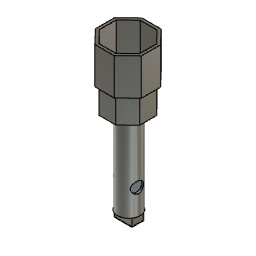
idea2 v1 (Autodesk Fusion 360 design; units mm, degrees)
Autodesk Fusion 360 part; units mm, degrees
sketch "Schizzo1" plane through (0, 0, 0) normal (0, 1, 0) x (1, 0, 0)
  line L0 (-15, -25) -> (15, -25)
  line L1 (15, -25) -> (37.4782, -5.1322)
  line L2 (37.4782, -5.1322) -> (37.4782, 24.8678)
  line L3 (37.4782, 24.8678) -> (15.4232, 45.2044)
  line L4 (15.4232, 45.2044) -> (-14.5768, 45.2044)
  line L5 (-14.5768, 45.2044) -> (-36.6318, 24.8678)
  line L6 (-36.6318, 24.8678) -> (-36.6318, -5.1322)
  line L7 (-36.6318, -5.1322) -> (-14.5368, -25.4254)
  dimension "d1" = 30
  dimension "d2" = 30
  dimension "d3" = 30
  dimension "d4" = 30
  dimension "d5" = 30
  dimension "d6" = 30
  dimension "d7" = 30
  constraint horizontal L0
  constraint perpendicular L0 L2
  constraint perpendicular L2 L4
  constraint perpendicular L4 L6
  measures "d1" distance of L0.end L1.end
  measures "d2" distance of L1.end L2.end
  measures "d3" distance of L2.end L3.end
  measures "d4" distance of L3.end L4.end
  measures "d5" distance of L4.end L5.end
  measures "d6" distance of L5.end L6.end
  measures "d7" distance of L6.end L7.end
sketch "Schizzo2" plane through (0, 0, 0) normal (0, 0, 1) x (1, 0, 0)
  line L0 (-15, 25) -> (15, 25)
  line L1 (15, 25) -> (35.8202, 3.4009)
  line L2 (35.8202, 3.4009) -> (35.8202, -26.5991)
  line L3 (35.8202, -26.5991) -> (14.221, -47.4193)
  line L4 (14.221, -47.4193) -> (-15.779, -47.4193)
  line L5 (-15.779, -47.4193) -> (-36.5991, -25.8202)
  line L6 (-36.5991, -25.8202) -> (-36.5991, 4.1798)
  line L7 (-36.5991, 4.1798) -> (-15, 25)
  dimension "d10" = 30
  dimension "d11" = 30
  dimension "d12" = 30
  dimension "d13" = 30
  dimension "d14" = 30
  dimension "d15" = 30
  dimension "d16" = 30
  constraint horizontal L0
  constraint perpendicular L0 L2
  constraint perpendicular L1 L3
  constraint perpendicular L2 L4
  constraint perpendicular L3 L5
  constraint perpendicular L4 L6
  measures "d10" distance of L0.end L1.end
  measures "d11" distance of L1.end L2.end
  measures "d12" distance of L2.end L3.end
  measures "d13" distance of L3.end L4.end
  measures "d14" distance of L4.end L5.end
  measures "d15" distance of L5.end L6.end
  measures "d16" distance of L0.start L6.end
extrude "Estrusione2" add sketch "Schizzo2" along normal blind 110 makes body 1
ref_plane "Piano di lavoro1" through (-0.3895, -11.2096, 50) normal (0, 0, 1) x (1, 0, 0)
split "Dividi1" by plane through (-0.3895, -11.2096, 50) normal (0, 0, 1) bodies 1 makes body 2 at (4.4807, -23.2795, 110)
shell "Svuotamento1" thickness 5 outward yes removed faces 1 at (4.4807, -23.2795, 110) on bodies 2
sketch "Schizzo3" plane through (0, 0, 0) normal (0, 0, -1) x (1, 0, 0)
  line L0 (-36.5991, 25.8202) -> (-36.5991, -4.1798)
  line L1 (-36.5991, -4.1798) -> (-15, -25)
  line L2 (-15, -25) -> (15, -25)
  line L3 (15, -25) -> (35.8202, -3.4009)
  line L4 (35.8202, -3.4009) -> (35.8202, 26.5991)
  line L5 (35.8202, 26.5991) -> (14.221, 47.4193)
  line L6 (14.221, 47.4193) -> (-15.779, 47.4193)
  line L7 (-15.779, 47.4193) -> (-36.5991, 25.8202)
  circle A0 centre (0, 10) radius 20
  line L8 (-15.9422, 20.1296) -> (15.6473, 20.1296)
  line L9 (15.6473, 20.1296) -> (15.6473, -0.5686)
  line L10 (15.6473, -0.5686) -> (-15.9422, -0.5686)
  line L11 (-15.9422, -0.5686) -> (-15.9422, 20.1296)
  constraint horizontal L8
  constraint vertical L9
  constraint horizontal L10
  constraint vertical L11
extrude "Estrusione3" add sketch "Schizzo3" along normal blind 155 contours A0 bodies 1
hole "Foratura1" at (19.6962, -13.473, -110.0448) direction (-0.984808, 0.173648, 0) diameter 20 depth 10 tip angle 118 bodies 1
hole "Foratura2" at (-20, -10, -107.3203) direction (1, 0, 0) diameter 20 depth 10 tip angle 118 bodies 1
sketch "Schizzo4" plane through (0, 0.5686, 0) normal (0, -1, 0) x (1, 0, 0)
  line L0 (15.6473, 0) -> (-15.9422, 0)
  line L1 (-15.9422, 0) -> (-15.9422, -155)
  line L2 (-15.9422, -155) -> (15.6473, -155)
  line L3 (15.6473, -155) -> (15.6473, 0)
sketch "Schizzo5" plane through (0, 0.5686, 0) normal (0, -1, 0) x (1, 0, 0)
sketch "Schizzo6" plane through (0, 0, -155) normal (0, 0, -1) x (1, 0, 0)
  line L0 (15.6473, -0.5686) -> (-15.9422, -0.5686)
  line L1 (-15.9422, -0.5686) -> (-15.9422, 20.1296)
  line L2 (-15.9422, 20.1296) -> (15.6473, 20.1296)
  line L3 (15.6473, 20.1296) -> (15.6473, -0.5686)
  circle A0 centre (0, 10) radius 20
  line L4 (-15.9422, 20.1296) -> (15.6473, 20.1296)
  line L5 (15.6473, -0.5686) -> (-15.9422, -0.5686)
  constraint coincident L1.end L2.start
  constraint coincident L2.end L3.start
  constraint coincident L0.start L3.end
  constraint coincident L0.end L1.start
extrude "Estrusione4" add sketch "Schizzo6" along normal blind 15 separate body contours L0 L1 L2 L3 L4 L5 makes body 3
shell "Svuotamento2" thickness 1 removed faces 1 at (-5.4123, -13.2302, -155) on bodies 3
named bodies: "Corpo PCB con pulsante LED e di accensione", "Corpo racchetta", "tappo"
